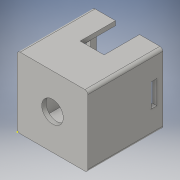
# Autodesk Inventor part: buttonInchPipeMount
Saved by Autodesk Inventor 2016 (Build 200138000, 138)
## iProperties
Created: 2016-07-21
Part Number: buttonInchPipeMount
Material: Generic
Document SubType Name: Modeling
Designer: cutrones
Density: 1 g/cm^3
Appearance: Default
Author: cutrones
Autodesk Inventor part; units mm, degrees
ref_plane "YZ Plane" through (0, 0, 0) normal (1, 0, 0) x (0, 1, 0)
ref_plane "XZ Plane" through (0, 0, 0) normal (0, 1, 0) x (-1, 0, 0)
ref_plane "XY Plane" through (0, 0, 0) normal (0, 0, 1) x (1, 0, 0)
sketch "Sketch1" plane through (0, 0, 0) normal (0, 0, 1) x (1, 0, 0)
  line L0 (0, 0) -> (76.2, 0)
  line L1 (76.2, 0) -> (76.2, 76.2)
  line L2 (76.2, 76.2) -> (0, 76.2)
  line L3 (0, 76.2) -> (0, 0)
  dimension "d0" = 76.2
  dimension "d1" = 76.2
  constraints: 8 end point, 2 parallel, 1 horizontal, 1 perpendicular
  measures "d0" distance of L2.end L1.end
  measures "d1" distance of L2.end L0.start
extrude "Extrusion1" add sketch "Sketch1" along normal blind 4.699
sketch "Sketch2" plane through (0, 0, 4.699) normal (0, 0, 1) x (1, 0, 0)
  point P0 (0, 0)
sketch "Sketch3" plane through (0, 0, 4.699) normal (0, 0, 1) x (1, 0, 0)
  circle A0 centre (38.1, 38.1) radius 11.6205
  line L0 (0, 76.2) -> (0, 0) projected
  line L1 (0, 0) -> (76.2, 0) projected
  point P0 (0, 73.025)
  point P1 (0, 3.175)
  point P2 (3.175, 0)
  point P3 (73.025, 0)
  dimension "d5" = 23.241
  dimension "d6" = 38.1
  dimension "d7" = 38.1
  constraints: 1 centre point
  measures "d5" diameter of A0
  measures "d6" distance from line of L0 A0.centre
  measures "d7" distance from line of L1 A0.centre
extrude "Extrusion2" cut sketch "Sketch3" against normal blind 4.699
sketch "Sketch5" plane through (0, 0, 0) normal (0, 0, -1) x (-1, 0, 0)
  line L0 (-4.699, 4.699) -> (-71.501, 4.699)
  line L1 (-71.501, 4.699) -> (-71.501, 71.501)
  line L2 (-71.501, 71.501) -> (-4.699, 71.501)
  line L3 (-4.699, 71.501) -> (-4.699, 4.699)
  line L4 (0, 0) -> (-76.2, 0) projected
  line L5 (0, 76.2) -> (0, 0) projected
  line L6 (-76.2, 76.2) -> (0, 76.2) projected
  line L7 (-76.2, 0) -> (-76.2, 76.2) projected
  line L8 (0, 76.2) -> (0, 0) projected
  line L9 (0, 0) -> (-76.2, 0)
  line L10 (-76.2, 0) -> (-76.2, 76.2)
  line L11 (-76.2, 76.2) -> (0, 76.2)
  line L12 (0, 76.2) -> (0, 0)
  dimension "d18" = 4.699
  dimension "d19" = 4.699
  dimension "d20" = 4.699
  dimension "d21" = 4.699
  constraints: 16 end point, 4 parallel, 2 horizontal, 2 perpendicular
  measures "d18" distance between parallel lines of L4 L0
  measures "d19" distance between parallel lines of L5 L3
  measures "d20" distance between parallel lines of L6 L2
  measures "d21" distance between parallel lines of L7 L1
extrude "Extrusion4" add sketch "Sketch5" along normal blind 76.2
sketch "Sketch6" plane through (0, 0, 4.699) normal (0, -1, 0) x (1, 0, 0)
  line L0 (4.699, -80.899) -> (71.501, -80.899) projected
  line L1 (25.146, -80.899) -> (51.054, -80.899)
  line L2 (51.054, -80.899) -> (51.054, -42.7482)
  line L3 (51.054, -42.7482) -> (25.146, -42.7482)
  line L4 (25.146, -42.7482) -> (25.146, -80.899)
  line L5 (76.2, -80.899) -> (76.2, 0) projected
  line L6 (0, 0) -> (0, -80.899) projected
  point P0 (0, -4.699)
  dimension "d24" = 25.908
  dimension "d25" = 38.1508
  dimension "d26" = 25.146
  dimension "d27" = 25.146
  constraints: 8 end point, 2 parallel, 1 horizontal, 1 perpendicular, 1 point on line
  measures "d24" distance of L2.end L3.end
  measures "d25" distance of L3.end L1.start
  measures "d26" distance between parallel lines of L5 L2
  measures "d27" distance between parallel lines of L6 L4
extrude "Extrusion5" cut sketch "Sketch6" against normal through all
sketch "Sketch7" plane through (76.2, 0, 4.699) normal (1, 0, 0) x (0, 0, -1)
  line L0 (74.549, 25.4) -> (68.199, 25.4)
  line L1 (68.199, 25.4) -> (68.199, 50.8)
  line L2 (68.199, 50.8) -> (74.549, 50.8)
  line L3 (74.549, 50.8) -> (74.549, 25.4)
  line L4 (80.899, 76.2) -> (80.899, 0) projected
  line L5 (80.899, 76.2) -> (0, 76.2) projected
  line L6 (80.899, 0) -> (0, 0) projected
  point P0 (4.699, 0)
  dimension "d30" = 6.35
  dimension "d31" = 25.4
  dimension "d32" = 6.35
  dimension "d33" = 25.4
  dimension "d34" = 25.4
  constraints: 8 end point, 2 parallel, 1 horizontal, 1 perpendicular
  measures "d30" distance of L1.end L2.end
  measures "d31" distance of L0.end L1.end
  measures "d32" distance between parallel lines of L4 L3
  measures "d33" distance between parallel lines of L5 L2
  measures "d34" distance between parallel lines of L6 L0
extrude "Extrusion6" cut sketch "Sketch7" against normal through all
fillet "Fillet2" radius 3.175 4 edges at (76.2, 76.2, -35.7505) (0, 76.2, -35.7505) (76.2, 0, -35.7505) (0, 0, -35.7505)
body "Solid1"
